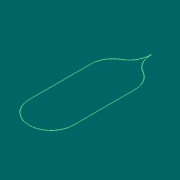
# Autodesk Inventor part: Fiber Loop
Saved by Autodesk Inventor 2016 (Build 200138000, 138)
## iProperties
Created: 2015-08-17
Part Number: Fiber Loop
Material: Glass
Document SubType Name: Modeling
Designer: Cosmic
Density: 2.18 g/cm^3
Appearance: Clear - Green 1
Author: Cosmic
Autodesk Inventor part; units mm, degrees
ref_plane "YZ Plane" through (0, 0, 0) normal (1, 0, 0) x (0, 1, 0)
ref_plane "XZ Plane" through (0, 0, 0) normal (0, 1, 0) x (-1, 0, 0)
ref_plane "XY Plane" through (0, 0, 0) normal (0, 0, 1) x (1, 0, 0)
sketch "Sketch1" plane through (0, 0, 0) normal (0, 0, 1) x (1, 0, 0)
  arc A0 (1.3, 83.7801) -> (24.5104, 44.4958) centre (46.15, 83.7801) ccw
  line L0 (-49.5, 0) -> (-49.5, -140)
  line L1 (49.5, 0) -> (49.5, -140)
  line L2 (0, 0) -> (0, -140)
  line L3 (-1.3, 83.7801) -> (1.3, 83.7801)
  arc A1 (49.5, 0) -> (23.8832, 43.3572) centre (0, 0) ccw
  arc A2 (-49.5, -140) -> (49.5, -140) centre (0, -140) ccw
  line L4 (-50.8, -140) -> (-50.8, 0)
  arc A3 (50.8, 0) -> (49.5, 11.4188) centre (0, 0) ccw
  line L5 (50.8, 0) -> (50.8, -140)
  arc A4 (-50.8, -140) -> (50.8, -140) centre (0, -140) ccw
  arc A5 (-17.7034, 47.4554) -> (-17.328, 47.7533) centre (-46.2999, 83.8687) ccw
  line L6 (0, 83.7801) -> (0, 0)
  line L7 (-50.65, 0) -> (-50.65, -140)
  arc A6 (-50.65, -140) -> (50.65, -140) centre (0, -140) ccw
  line L8 (50.65, -140) -> (50.65, 0)
  arc A7 (50.65, 0) -> (49.5, 10.7318) centre (0, 0) ccw
  line L9 (-49.65, 0) -> (-49.65, -140)
  arc A8 (-49.65, -140) -> (49.65, -140) centre (0, -140) ccw
  line L10 (49.65, -140) -> (49.65, 0)
  arc A9 (49.65, 0) -> (49.5, 3.8565) centre (0, 0) ccw
  arc A10 (-18.1806, 47.2746) -> (-17.7777, 47.5877) centre (-46.2999, 83.8687) ccw
  arc A11 (-24.479, 44.3418) -> (-22.1739, 45.7051) centre (-46.2999, 83.8687) ccw
  arc A12 (-23.9232, 43.3351) -> (-49.5, 0) centre (0, 0) ccw
  arc A13 (-26.3069, 42.1078) -> (-49.5, 3.8565) centre (0, 0) ccw
  arc A14 (-23.9957, 43.4664) -> (-26.3069, 42.1078) centre (0, 0) ccw
  arc A15 (-23.9957, 43.4664) -> (-18.1806, 47.2746) centre (-46.2999, 83.8687) ccw
  arc A16 (-21.6146, 44.6982) -> (-17.7034, 47.4554) centre (-46.2999, 83.8687) ccw
  arc A17 (-24.479, 44.3418) -> (-30.3169, 40.5747) centre (0, 0) ccw
  arc A18 (-24.5515, 44.4732) -> (-1.3, 83.7801) centre (-46.2999, 83.8687) ccw
  arc A19 (-24.5515, 44.4732) -> (-26.8609, 43.1176) centre (0, 0) ccw
  arc A20 (-30.3169, 40.5747) -> (-50.65, 0) centre (0, 0) ccw
  arc A21 (-26.8609, 43.1176) -> (-30.7965, 40.4007) centre (0, 0) ccw
  arc A22 (-30.7965, 40.4007) -> (-50.8, 0) centre (0, 0) ccw
  arc A23 (-49.5, 3.8565) -> (-49.65, 0) centre (0, 0) ccw
  arc A24 (-23.9232, 43.3351) -> (-21.6146, 44.6982) centre (-46.2999, 83.8687) ccw
  arc A25 (-17.7777, 47.5877) -> (-0.15, 83.7801) centre (-46.2999, 83.8687) ccw
  arc A26 (-22.1739, 45.7051) -> (-1.15, 83.7801) centre (-46.2999, 83.8687) ccw
  arc A27 (26.3069, 42.1078) -> (23.9556, 43.4886) centre (0, 0) ccw
  arc A28 (26.819, 43.1437) -> (24.5104, 44.4958) centre (0, 0) ccw
  arc A29 (30.754, 40.4331) -> (26.819, 43.1437) centre (0, 0) ccw
  arc A30 (22.1042, 45.7433) -> (24.438, 44.3645) centre (46.15, 83.7801) ccw
  arc A31 (1.15, 83.7801) -> (22.1042, 45.7433) centre (46.15, 83.7801) ccw
  arc A32 (17.2904, 47.767) -> (17.6461, 47.4847) centre (46.15, 83.7801) ccw
  arc A33 (17.6461, 47.4847) -> (21.5447, 44.7365) centre (46.15, 83.7801) ccw
  arc A34 (21.5447, 44.7365) -> (23.8832, 43.3572) centre (46.15, 83.7801) ccw
  arc A35 (18.1221, 47.3049) -> (23.9556, 43.4886) centre (46.15, 83.7801) ccw
  arc A36 (49.5, 3.8565) -> (26.3069, 42.1078) centre (0, 0) ccw
  arc A37 (30.3169, 40.5747) -> (24.438, 44.3645) centre (0, 0) ccw
  arc A38 (0, 83.8243) -> (17.2904, 47.767) centre (46.15, 83.7801) ccw
  arc A39 (17.7205, 47.617) -> (18.1221, 47.3049) centre (46.15, 83.7801) ccw
  arc A40 (0.15, 83.7801) -> (17.7205, 47.617) centre (46.15, 83.7801) ccw
  arc A41 (31.1763, 40.1084) -> (30.754, 40.4331) centre (0, 0) ccw
  arc A42 (49.5, 11.4188) -> (31.1763, 40.1084) centre (0, 0) ccw
  arc A43 (30.7241, 40.2673) -> (30.3169, 40.5747) centre (0, 0) ccw
  arc A44 (49.5, 10.7318) -> (30.7241, 40.2673) centre (0, 0) ccw
  arc A45 (-17.328, 47.7533) -> (0, 83.8243) centre (-46.2999, 83.8687) ccw
  dimension "d44" = 140
  dimension "d45" = 49.5
  dimension "d48" = 1.3
  dimension "d49" = 0.15
  dimension "d50" = 0.15
  dimension "d53" = 0.15
  dimension "d55" = 0.15
  dimension "d56" = 0.15
  dimension "d57" = 1.3
  dimension "d58" = 1.3
  dimension "d61" = 45
  dimension "d62" = 1.3
  dimension "d63" = 1.3
  dimension "d64" = 1.3
  dimension "d65" = 0.15
  dimension "d66" = 0.15
  dimension "d67" = 45
  constraints: 107 point on circle, 46 centre point, 22 end point, 12 tangent, 9 point on line, 4 parallel, 2 midpoint, 1 coincident, 1 horizontal, 1 line through centre, 1 perpendicular, 1 vertical, 6 other
  measures "d44" distance of L2.start L2.end
  measures "d45" radius of A1
  measures "d48" radial gap between concentric circles of A3 A1
  measures "d49" radial gap between concentric circles of A3 A7
  measures "d50" radial gap between concentric circles of A1 A9
  measures "d53" radial gap between concentric circles of A10 A5
  measures "d55" distance between parallel lines of L10 L1
  measures "d56" distance between parallel lines of L5 L8
  measures "d57" distance between parallel lines of L1 L5
  measures "d58" distance between parallel lines of L0 L4
  measures "d61" radius of A18
  measures "d62" radial gap between concentric circles of A22 A12
  measures "d63" radial gap between concentric circles of A0 A38
  measures "d64" radial gap between concentric circles of A18 A45
  measures "d65" radial gap between concentric circles of A22 A20
  measures "d66" radial gap between concentric circles of A12 A23
  measures "d67" radius of A31
extrude "Extrusion3" add sketch "Sketch1" along normal blind 1 contours A31 A30 A37 A43 A44 A7 L8 A6 L7 A20 A17 A11 A26 L3 A25 A10 A15 A14 A13 A23 L9 A8 L10 A9 A36 A27 A35 A39 A40
sketch "Sketch3" plane through (-1.15, 83.7801, 0) normal (0, 1, 0) x (1, 0, 0)
  line L0 (2.3, 0) -> (1.3, 0) projected
  line L1 (1.3, 0) -> (1.3, -1) projected
  line L2 (2.3, -1) -> (1.3, -1) projected
  line L3 (2.3, 0) -> (2.3, -1) projected
  line L4 (1, 0) -> (0, 0) projected
  line L5 (0, 0) -> (0, -1) projected
  line L6 (1, -1) -> (0, -1) projected
  line L7 (1, 0) -> (1, -1) projected
  point P0 (1.15, 0)
extrude "Extrusion4" add sketch "Sketch3" along normal blind 3
fillet "Fillet2" radius 0.495 36 edges at (6.5461, 60.3808, 0) (42.7464, 25.256, 0) (49.65, -70, 0) (0, -189.65, 0) (-49.65, -70, 0) (-42.7581, 25.2362, 0) (-6.5785, 60.3733, 0) (0.15, 85.2801, 0) (-0.15, 85.2801, 0) (49.65, -70, 1) (0, -189.65, 1) (-49.65, -70, 1) (-42.7581, 25.2362, 1) (-6.5785, 60.3733, 1) (6.5461, 60.3808, 1) (0.15, 85.2801, 1) (42.7464, 25.256, 1) (-0.15, 85.2801, 1) (7.407, 60.8894, 0) (43.6074, 25.7647, 0) (50.65, -70, 0) (0, -190.65, 0) (-50.65, -70, 0) (-43.6193, 25.7445, 0) (-7.4397, 60.8816, 0) (1.15, 85.2801, 0) (7.407, 60.8894, 1) (43.6074, 25.7647, 1) (50.65, -70, 1) (0, -190.65, 1) (-50.65, -70, 1) (-43.6193, 25.7445, 1) (-7.4397, 60.8816, 1) (1.15, 85.2801, 1) (-1.15, 85.2801, 1) (-1.15, 85.2801, 0)
equation "\"d44\" = LoopLength"
equation "\"d48\" = OpticalFiberDiameter + 2 * OpticalFiberClearence"
equation "\"d49\" = OpticalFiberClearence"
equation "\"d50\" = OpticalFiberClearence"
equation "\"d53\" = OpticalFiberClearence"
equation "\"d55\" = OpticalFiberClearence"
equation "\"d56\" = OpticalFiberClearence"
equation "\"d57\" = OpticalFiberDiameter + 2 * OpticalFiberClearence"
equation "\"d58\" = OpticalFiberDiameter + 2 * OpticalFiberClearence"
equation "\"d61\" = 0.5 * LoopSmallTrackDiameter"
equation "\"d59\" = OpticalFiberDiameter"
equation "\"OpticalFiberDiameter\" = 1"
equation "\"OpticalFiberClearence\" = 0.15"
equation "\"ScintillatorEdgeClearence\" = 3"
equation "\"MPPCDepth\" = 1"
equation "\"LoopLargeTrackRatio\" = 1.1"
equation "\"d24\" = 0.05"
equation "\"d25\" = 1"
equation "\"d32\" = 0.05"
equation "\"d33\" = 1"
equation "\"FiberSensorClerence\" = 0.5"
equation "\"SmallTrackDiameter\" = 175"
equation "\"ScintillatorWidth\" = 145"
equation "\"ShallowTrackDepth\" = 1.3"
equation "\"MPPCClearence\" = 0.075"
equation "\"MPPCSensorClearence\" = 1.45"
equation "\"MPPCSensorOffsett\" = 2.105"
equation "\"MPPCWidth\" = 5.9"
equation "\"MPPCHeight\" = 6.55"
equation "\"FiberEdgeOffsett\" = 5"
equation "\"LongFiberAngle\" = 30deg"
equation "\"ShortFiberAngle\" = 78deg"
equation "\"MountingScrewOffsett\" = 12"
equation "\"MountingScrewDepth\" = 2"
equation "\"LoopLength\" = 140"
equation "\"d46\" = OpticalFiberDiameter + 2 * OpticalFiberClearence"
equation "\"d54\" = OpticalFiberClearence"
equation "\"LoopSmallTrackDiameter\" = 90"
body "Solid1"
body "Solid2"
